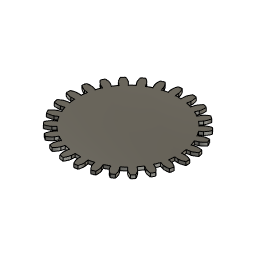
Gear1Finger (Autodesk Fusion 360 design; units mm, degrees)
Autodesk Fusion 360 part; units mm, degrees
sketch "Sketch1" plane through (0, 0, 0) normal (0, 0, 1) x (1, 0, 0)
  spline S0 degree 5 poles (2.4571, -0.2414) (2.4571, -0.2414) (2.4572, -0.2414) (2.4572, -0.2414) (2.4573, -0.2414) (2.4574, -0.2415) (2.4575, -0.2415) (2.4577, -0.2415) (2.4578, -0.2415) (2.458, -0.2415) (2.4582, -0.2415) (2.4584, -0.2415) (2.4586, -0.2415) (2.4589, -0.2416) (2.4591, -0.2416) (2.4594, -0.2416) (2.4597, -0.2416) (2.46, -0.2416) (2.4603, -0.2416) (2.4606, -0.2416) (2.461, -0.2417) (2.4614, -0.2417) (2.4617, -0.2417) (2.4621, -0.2417) (2.4625, -0.2417) (2.463, -0.2417) (2.4634, -0.2417) (2.4639, -0.2417) (2.4643, -0.2418) (2.4648, -0.2418) (2.4653, -0.2418) (2.4658, -0.2418) (2.4664, -0.2418) (2.4669, -0.2418) (2.4675, -0.2418) (2.4681, -0.2418) (2.4686, -0.2418) (2.4692, -0.2418) (2.4699, -0.2418) (2.4705, -0.2418) (2.4712, -0.2418) (2.4718, -0.2418) (2.4725, -0.2418) (2.4732, -0.2418) (2.4739, -0.2418) (2.4746, -0.2417) (2.4754, -0.2417) (2.4761, -0.2417) (2.4769, -0.2417) (2.4777, -0.2417) (2.4785, -0.2416) (2.4793, -0.2416) (2.4801, -0.2416) (2.4809, -0.2415) (2.4818, -0.2415) (2.4826, -0.2415) (2.4835, -0.2414) (2.4844, -0.2414) (2.4853, -0.2413) (2.4862, -0.2413) (2.4872, -0.2412) (2.4881, -0.2412) (2.4891, -0.2411) (2.4901, -0.241) (2.4911, -0.241) (2.4921, -0.2409) (2.4931, -0.2408) (2.4941, -0.2408) (2.4952, -0.2407) (2.4962, -0.2406) (2.4973, -0.2405) (2.4984, -0.2404) (2.4995, -0.2403) (2.5006, -0.2402) (2.5017, -0.2401) (2.5029, -0.24) (2.504, -0.2399) (2.5052, -0.2398) (2.5064, -0.2397) (2.5076, -0.2395) (2.5088, -0.2394) (2.51, -0.2393) (2.5112, -0.2391) (2.5125, -0.239) (2.5137, -0.2388) (2.515, -0.2387) (2.5163, -0.2385) (2.5176, -0.2384) (2.5189, -0.2382) (2.5202, -0.238) (2.5216, -0.2379) (2.5229, -0.2377) (2.5243, -0.2375) (2.5256, -0.2373) (2.527, -0.2371) (2.5284, -0.2369) (2.5298, -0.2367) (2.5313, -0.2365) (2.5327, -0.2363) (2.5341, -0.2361) (2.5356, -0.2358) (2.5371, -0.2356) (2.5386, -0.2354) (2.5401, -0.2351) (2.5416, -0.2349) (2.5431, -0.2346) (2.5446, -0.2344) (2.5462, -0.2341) (2.5477, -0.2338) (2.5493, -0.2336) (2.5509, -0.2333) (2.5525, -0.233) (2.5541, -0.2327) (2.5557, -0.2324) (2.5573, -0.2321) (2.559, -0.2318) (2.5606, -0.2314) (2.5623, -0.2311) (2.564, -0.2308) (2.5657, -0.2304) (2.5674, -0.2301) (2.5691, -0.2297) (2.5708, -0.2294) (2.5725, -0.229) (2.5743, -0.2286) (2.576, -0.2283) (2.5778, -0.2279) (2.5796, -0.2275) (2.5814, -0.2271) (2.5832, -0.2267) (2.585, -0.2263) (2.5868, -0.2258) (2.5886, -0.2254) (2.5905, -0.225) (2.5923, -0.2245) (2.5942, -0.2241) (2.5961, -0.2236) (2.598, -0.2232) (2.5999, -0.2227) (2.6018, -0.2222) (2.6037, -0.2217) (2.6056, -0.2212) (2.6076, -0.2207) (2.6095, -0.2202) (2.6115, -0.2197) (2.6135, -0.2192) (2.6154, -0.2187) (2.6174, -0.2181) (2.6194, -0.2176) (2.6214, -0.217) (2.6235, -0.2165) (2.6255, -0.2159) (2.6275, -0.2153) (2.6296, -0.2147) (2.6317, -0.2141) (2.6337, -0.2135) (2.6358, -0.2129) (2.6379, -0.2123) (2.64, -0.2117) (2.6421, -0.211) (2.6443, -0.2104) (2.6464, -0.2097) (2.6485, -0.2091) (2.6507, -0.2084) (2.6528, -0.2077) (2.655, -0.2071) (2.6572, -0.2064) (2.6594, -0.2057) (2.6616, -0.2049) (2.6638, -0.2042) (2.666, -0.2035) (2.6682, -0.2028) (2.6705, -0.202) (2.6727, -0.2013) (2.675, -0.2005) (2.6772, -0.1997) (2.6795, -0.199) (2.6818, -0.1982) (2.6841, -0.1974) (2.6864, -0.1966) (2.6887, -0.1957) (2.691, -0.1949) (2.6933, -0.1941) (2.6957, -0.1932) (2.698, -0.1924) (2.7004, -0.1915) (2.7027, -0.1907) (2.7051, -0.1898) (2.7075, -0.1889) (2.7099, -0.188) (2.7123, -0.1871) (2.7147, -0.1862) (2.7171, -0.1852) (2.7195, -0.1843) (2.7219, -0.1834) (2.7244, -0.1824) (2.7268, -0.1815) (2.7293, -0.1805) (2.7317, -0.1795) (2.7342, -0.1785) (2.7367, -0.1775) (2.7391, -0.1765) (2.7416, -0.1755) (2.7441, -0.1744) (2.7466, -0.1734) (2.7492, -0.1723) (2.7517, -0.1713) (2.7542, -0.1702) (2.7567, -0.1691) (2.7593, -0.168) (2.7618, -0.1669) (2.7644, -0.1658) (2.767, -0.1647) (2.7695, -0.1636) (2.7721, -0.1624) (2.7747, -0.1613) (2.7773, -0.1601) (2.7799, -0.159) (2.7825, -0.1578) (2.7851, -0.1566) (2.7878, -0.1554) (2.7904, -0.1542) (2.793, -0.153) (2.7957, -0.1517) (2.7983, -0.1505) (2.801, -0.1492) (2.8037, -0.148) (2.8063, -0.1467) (2.809, -0.1454) (2.8117, -0.1441) (2.8144, -0.1428) (2.8171, -0.1415) (2.8198, -0.1402) (2.8225, -0.1388) (2.8252, -0.1375) (2.828, -0.1361) (2.8307, -0.1348) (2.8334, -0.1334) (2.8362, -0.132) (2.8389, -0.1306) (2.8417, -0.1292) (2.8439, -0.128) (2.8455, -0.1272) (2.8466, -0.1266) (2.8472, -0.1263) knots 0 0 0 0 0 0 0.00416667 0.00833333 0.0125 0.01666667 0.02083333 0.025 0.02916667 0.03333333 0.0375 0.04166667 0.04583333 0.05 0.05416667 0.05833333 0.0625 0.06666667 0.07083333 0.075 0.07916667 0.08333333 0.0875 0.09166667 0.09583333 0.1 0.10416667 0.10833333 0.1125 0.11666667 0.12083333 0.125 0.12916667 0.13333333 0.1375 0.14166667 0.14583333 0.15 0.15416667 0.15833333 0.1625 0.16666667 0.17083333 0.175 0.17916667 0.18333333 0.1875 0.19166667 0.19583333 0.2 0.20416667 0.20833333 0.2125 0.21666667 0.22083333 0.225 0.22916667 0.23333333 0.2375 0.24166667 0.24583333 0.25 0.25416667 0.25833333 0.2625 0.26666667 0.27083333 0.275 0.27916667 0.28333333 0.2875 0.29166667 0.29583333 0.3 0.30416667 0.30833333 0.3125 0.31666667 0.32083333 0.325 0.32916667 0.33333333 0.3375 0.34166667 0.34583333 0.35 0.35416667 0.35833333 0.3625 0.36666667 0.37083333 0.375 0.37916667 0.38333333 0.3875 0.39166667 0.39583333 0.4 0.40416667 0.40833333 0.4125 0.41666667 0.42083333 0.425 0.42916667 0.43333333 0.4375 0.44166667 0.44583333 0.45 0.45416667 0.45833333 0.4625 0.46666667 0.47083333 0.475 0.47916667 0.48333333 0.4875 0.49166667 0.49583333 0.5 0.50416667 0.50833333 0.5125 0.51666667 0.52083333 0.525 0.52916667 0.53333333 0.5375 0.54166667 0.54583333 0.55 0.55416667 0.55833333 0.5625 0.56666667 0.57083333 0.575 0.57916667 0.58333333 0.5875 0.59166667 0.59583333 0.6 0.60416667 0.60833333 0.6125 0.61666667 0.62083333 0.625 0.62916667 0.63333333 0.6375 0.64166667 0.64583333 0.65 0.65416667 0.65833333 0.6625 0.66666667 0.67083333 0.675 0.67916667 0.68333333 0.6875 0.69166667 0.69583333 0.7 0.70416667 0.70833333 0.7125 0.71666667 0.72083333 0.725 0.72916667 0.73333333 0.7375 0.74166667 0.74583333 0.75 0.75416667 0.75833333 0.7625 0.76666667 0.77083333 0.775 0.77916667 0.78333333 0.7875 0.79166667 0.79583333 0.8 0.80416667 0.80833333 0.8125 0.81666667 0.82083333 0.825 0.82916667 0.83333333 0.8375 0.84166667 0.84583333 0.85 0.85416667 0.85833333 0.8625 0.86666667 0.87083333 0.875 0.87916667 0.88333333 0.8875 0.89166667 0.89583333 0.9 0.90416667 0.90833333 0.9125 0.91666667 0.92083333 0.925 0.92916667 0.93333333 0.9375 0.94166667 0.94583333 0.95 0.95416667 0.95833333 0.9625 0.96666667 0.97083333 0.975 0.97916667 0.98333333 0.9875 0.99166667 0.99583333 1 1 1 1 1 1
  spline S1 degree 5 poles (2.4571, 0.2414) (2.4571, 0.2414) (2.4572, 0.2414) (2.4572, 0.2414) (2.4573, 0.2414) (2.4574, 0.2415) (2.4575, 0.2415) (2.4577, 0.2415) (2.4578, 0.2415) (2.458, 0.2415) (2.4582, 0.2415) (2.4584, 0.2415) (2.4586, 0.2415) (2.4589, 0.2416) (2.4591, 0.2416) (2.4594, 0.2416) (2.4597, 0.2416) (2.46, 0.2416) (2.4603, 0.2416) (2.4606, 0.2416) (2.461, 0.2417) (2.4614, 0.2417) (2.4617, 0.2417) (2.4621, 0.2417) (2.4625, 0.2417) (2.463, 0.2417) (2.4634, 0.2417) (2.4639, 0.2417) (2.4643, 0.2418) (2.4648, 0.2418) (2.4653, 0.2418) (2.4658, 0.2418) (2.4664, 0.2418) (2.4669, 0.2418) (2.4675, 0.2418) (2.4681, 0.2418) (2.4686, 0.2418) (2.4692, 0.2418) (2.4699, 0.2418) (2.4705, 0.2418) (2.4712, 0.2418) (2.4718, 0.2418) (2.4725, 0.2418) (2.4732, 0.2418) (2.4739, 0.2418) (2.4746, 0.2417) (2.4754, 0.2417) (2.4761, 0.2417) (2.4769, 0.2417) (2.4777, 0.2417) (2.4785, 0.2416) (2.4793, 0.2416) (2.4801, 0.2416) (2.4809, 0.2415) (2.4818, 0.2415) (2.4826, 0.2415) (2.4835, 0.2414) (2.4844, 0.2414) (2.4853, 0.2413) (2.4862, 0.2413) (2.4872, 0.2412) (2.4881, 0.2412) (2.4891, 0.2411) (2.4901, 0.241) (2.4911, 0.241) (2.4921, 0.2409) (2.4931, 0.2408) (2.4941, 0.2408) (2.4952, 0.2407) (2.4962, 0.2406) (2.4973, 0.2405) (2.4984, 0.2404) (2.4995, 0.2403) (2.5006, 0.2402) (2.5017, 0.2401) (2.5029, 0.24) (2.504, 0.2399) (2.5052, 0.2398) (2.5064, 0.2397) (2.5076, 0.2395) (2.5088, 0.2394) (2.51, 0.2393) (2.5112, 0.2391) (2.5125, 0.239) (2.5137, 0.2388) (2.515, 0.2387) (2.5163, 0.2385) (2.5176, 0.2384) (2.5189, 0.2382) (2.5202, 0.238) (2.5216, 0.2379) (2.5229, 0.2377) (2.5243, 0.2375) (2.5256, 0.2373) (2.527, 0.2371) (2.5284, 0.2369) (2.5298, 0.2367) (2.5313, 0.2365) (2.5327, 0.2363) (2.5341, 0.2361) (2.5356, 0.2358) (2.5371, 0.2356) (2.5386, 0.2354) (2.5401, 0.2351) (2.5416, 0.2349) (2.5431, 0.2346) (2.5446, 0.2344) (2.5462, 0.2341) (2.5477, 0.2338) (2.5493, 0.2336) (2.5509, 0.2333) (2.5525, 0.233) (2.5541, 0.2327) (2.5557, 0.2324) (2.5573, 0.2321) (2.559, 0.2318) (2.5606, 0.2314) (2.5623, 0.2311) (2.564, 0.2308) (2.5657, 0.2304) (2.5674, 0.2301) (2.5691, 0.2297) (2.5708, 0.2294) (2.5725, 0.229) (2.5743, 0.2286) (2.576, 0.2283) (2.5778, 0.2279) (2.5796, 0.2275) (2.5814, 0.2271) (2.5832, 0.2267) (2.585, 0.2263) (2.5868, 0.2258) (2.5886, 0.2254) (2.5905, 0.225) (2.5923, 0.2245) (2.5942, 0.2241) (2.5961, 0.2236) (2.598, 0.2232) (2.5999, 0.2227) (2.6018, 0.2222) (2.6037, 0.2217) (2.6056, 0.2212) (2.6076, 0.2207) (2.6095, 0.2202) (2.6115, 0.2197) (2.6135, 0.2192) (2.6154, 0.2187) (2.6174, 0.2181) (2.6194, 0.2176) (2.6214, 0.217) (2.6235, 0.2165) (2.6255, 0.2159) (2.6275, 0.2153) (2.6296, 0.2147) (2.6317, 0.2141) (2.6337, 0.2135) (2.6358, 0.2129) (2.6379, 0.2123) (2.64, 0.2117) (2.6421, 0.211) (2.6443, 0.2104) (2.6464, 0.2097) (2.6485, 0.2091) (2.6507, 0.2084) (2.6528, 0.2077) (2.655, 0.2071) (2.6572, 0.2064) (2.6594, 0.2057) (2.6616, 0.2049) (2.6638, 0.2042) (2.666, 0.2035) (2.6682, 0.2028) (2.6705, 0.202) (2.6727, 0.2013) (2.675, 0.2005) (2.6772, 0.1997) (2.6795, 0.199) (2.6818, 0.1982) (2.6841, 0.1974) (2.6864, 0.1966) (2.6887, 0.1957) (2.691, 0.1949) (2.6933, 0.1941) (2.6957, 0.1932) (2.698, 0.1924) (2.7004, 0.1915) (2.7027, 0.1907) (2.7051, 0.1898) (2.7075, 0.1889) (2.7099, 0.188) (2.7123, 0.1871) (2.7147, 0.1862) (2.7171, 0.1852) (2.7195, 0.1843) (2.7219, 0.1834) (2.7244, 0.1824) (2.7268, 0.1815) (2.7293, 0.1805) (2.7317, 0.1795) (2.7342, 0.1785) (2.7367, 0.1775) (2.7391, 0.1765) (2.7416, 0.1755) (2.7441, 0.1744) (2.7466, 0.1734) (2.7492, 0.1723) (2.7517, 0.1713) (2.7542, 0.1702) (2.7567, 0.1691) (2.7593, 0.168) (2.7618, 0.1669) (2.7644, 0.1658) (2.767, 0.1647) (2.7695, 0.1636) (2.7721, 0.1624) (2.7747, 0.1613) (2.7773, 0.1601) (2.7799, 0.159) (2.7825, 0.1578) (2.7851, 0.1566) (2.7878, 0.1554) (2.7904, 0.1542) (2.793, 0.153) (2.7957, 0.1517) (2.7983, 0.1505) (2.801, 0.1492) (2.8037, 0.148) (2.8063, 0.1467) (2.809, 0.1454) (2.8117, 0.1441) (2.8144, 0.1428) (2.8171, 0.1415) (2.8198, 0.1402) (2.8225, 0.1388) (2.8252, 0.1375) (2.828, 0.1361) (2.8307, 0.1348) (2.8334, 0.1334) (2.8362, 0.132) (2.8389, 0.1306) (2.8417, 0.1292) (2.8439, 0.128) (2.8455, 0.1272) (2.8466, 0.1266) (2.8472, 0.1263) knots 0 0 0 0 0 0 0.00416667 0.00833333 0.0125 0.01666667 0.02083333 0.025 0.02916667 0.03333333 0.0375 0.04166667 0.04583333 0.05 0.05416667 0.05833333 0.0625 0.06666667 0.07083333 0.075 0.07916667 0.08333333 0.0875 0.09166667 0.09583333 0.1 0.10416667 0.10833333 0.1125 0.11666667 0.12083333 0.125 0.12916667 0.13333333 0.1375 0.14166667 0.14583333 0.15 0.15416667 0.15833333 0.1625 0.16666667 0.17083333 0.175 0.17916667 0.18333333 0.1875 0.19166667 0.19583333 0.2 0.20416667 0.20833333 0.2125 0.21666667 0.22083333 0.225 0.22916667 0.23333333 0.2375 0.24166667 0.24583333 0.25 0.25416667 0.25833333 0.2625 0.26666667 0.27083333 0.275 0.27916667 0.28333333 0.2875 0.29166667 0.29583333 0.3 0.30416667 0.30833333 0.3125 0.31666667 0.32083333 0.325 0.32916667 0.33333333 0.3375 0.34166667 0.34583333 0.35 0.35416667 0.35833333 0.3625 0.36666667 0.37083333 0.375 0.37916667 0.38333333 0.3875 0.39166667 0.39583333 0.4 0.40416667 0.40833333 0.4125 0.41666667 0.42083333 0.425 0.42916667 0.43333333 0.4375 0.44166667 0.44583333 0.45 0.45416667 0.45833333 0.4625 0.46666667 0.47083333 0.475 0.47916667 0.48333333 0.4875 0.49166667 0.49583333 0.5 0.50416667 0.50833333 0.5125 0.51666667 0.52083333 0.525 0.52916667 0.53333333 0.5375 0.54166667 0.54583333 0.55 0.55416667 0.55833333 0.5625 0.56666667 0.57083333 0.575 0.57916667 0.58333333 0.5875 0.59166667 0.59583333 0.6 0.60416667 0.60833333 0.6125 0.61666667 0.62083333 0.625 0.62916667 0.63333333 0.6375 0.64166667 0.64583333 0.65 0.65416667 0.65833333 0.6625 0.66666667 0.67083333 0.675 0.67916667 0.68333333 0.6875 0.69166667 0.69583333 0.7 0.70416667 0.70833333 0.7125 0.71666667 0.72083333 0.725 0.72916667 0.73333333 0.7375 0.74166667 0.74583333 0.75 0.75416667 0.75833333 0.7625 0.76666667 0.77083333 0.775 0.77916667 0.78333333 0.7875 0.79166667 0.79583333 0.8 0.80416667 0.80833333 0.8125 0.81666667 0.82083333 0.825 0.82916667 0.83333333 0.8375 0.84166667 0.84583333 0.85 0.85416667 0.85833333 0.8625 0.86666667 0.87083333 0.875 0.87916667 0.88333333 0.8875 0.89166667 0.89583333 0.9 0.90416667 0.90833333 0.9125 0.91666667 0.92083333 0.925 0.92916667 0.93333333 0.9375 0.94166667 0.94583333 0.95 0.95416667 0.95833333 0.9625 0.96666667 0.97083333 0.975 0.97916667 0.98333333 0.9875 0.99166667 0.99583333 1 1 1 1 1 1
  spline S2 degree 5 poles (2.4569, -0.2414) (2.457, -0.2414) (2.457, -0.2414) (2.457, -0.2414) (2.457, -0.2414) (2.457, -0.2414) (2.4571, -0.2414) (2.4571, -0.2414) (2.4571, -0.2414) (2.4571, -0.2414) knots 0 0 0 0 0 0 0.2 0.4 0.6 0.8 1 1 1 1 1 1
  spline S3 degree 5 poles (2.4569, 0.2414) (2.457, 0.2414) (2.457, 0.2414) (2.457, 0.2414) (2.457, 0.2414) (2.457, 0.2414) (2.4571, 0.2414) (2.4571, 0.2414) (2.4571, 0.2414) (2.4571, 0.2414) knots 0 0 0 0 0 0 0.2 0.4 0.6 0.8 1 1 1 1 1 1
  line L0 (0, 0) -> (2.4569, -0.2414)
  line L1 (0, 0) -> (2.4569, 0.2414)
  arc A0 (2.8472, -0.1263) -> (2.8472, 0.1263) centre (0, 0) ccw
  point P0 (2.4576, -0.2415)
  point P1 (2.4585, -0.2415)
  point P2 (2.4597, -0.2416)
  point P3 (2.4612, -0.2417)
  point P4 (2.4631, -0.2417)
  point P5 (2.4653, -0.2418)
  point P6 (2.4679, -0.2418)
  point P7 (2.4708, -0.2418)
  point P8 (2.474, -0.2417)
  point P9 (2.4776, -0.2417)
  point P10 (2.4816, -0.2415)
  point P11 (2.4858, -0.2413)
  point P12 (2.4904, -0.241)
  point P13 (2.4954, -0.2407)
  point P14 (2.5007, -0.2402)
  point P15 (2.5063, -0.2397)
  point P16 (2.5122, -0.239)
  point P17 (2.5185, -0.2383)
  point P18 (2.5251, -0.2374)
  point P19 (2.5321, -0.2364)
  point P20 (2.5393, -0.2352)
  point P21 (2.5469, -0.234)
  point P22 (2.5548, -0.2325)
  point P23 (2.5631, -0.231)
  point P24 (2.5716, -0.2292)
  point P25 (2.5805, -0.2273)
  point P26 (2.5896, -0.2252)
  point P27 (2.5991, -0.2229)
  point P28 (2.6089, -0.2204)
  point P29 (2.619, -0.2177)
  point P30 (2.6294, -0.2148)
  point P31 (2.64, -0.2117)
  point P32 (2.651, -0.2083)
  point P33 (2.6622, -0.2047)
  point P34 (2.6738, -0.2009)
  point P35 (2.6856, -0.1969)
  point P36 (2.6976, -0.1925)
  point P37 (2.71, -0.188)
  point P38 (2.7226, -0.1831)
  point P39 (2.7355, -0.178)
  point P40 (2.7486, -0.1726)
  point P41 (2.762, -0.1669)
  point P42 (2.7756, -0.1609)
  point P43 (2.7895, -0.1546)
  point P44 (2.8036, -0.148)
  point P45 (2.8179, -0.1411)
  point P46 (2.8324, -0.1339)
  point P47 (2.4576, 0.2415)
  point P48 (2.4585, 0.2415)
  point P49 (2.4597, 0.2416)
  point P50 (2.4612, 0.2417)
  point P51 (2.4631, 0.2417)
  point P52 (2.4653, 0.2418)
  point P53 (2.4679, 0.2418)
  point P54 (2.4708, 0.2418)
  point P55 (2.474, 0.2417)
  point P56 (2.4776, 0.2417)
  point P57 (2.4816, 0.2415)
  point P58 (2.4858, 0.2413)
  point P59 (2.4904, 0.241)
  point P60 (2.4954, 0.2407)
  point P61 (2.5007, 0.2402)
  point P62 (2.5063, 0.2397)
  point P63 (2.5122, 0.239)
  point P64 (2.5185, 0.2383)
  point P65 (2.5251, 0.2374)
  point P66 (2.5321, 0.2364)
  point P67 (2.5393, 0.2352)
  point P68 (2.5469, 0.234)
  point P69 (2.5548, 0.2325)
  point P70 (2.5631, 0.231)
  point P71 (2.5716, 0.2292)
  point P72 (2.5805, 0.2273)
  point P73 (2.5896, 0.2252)
  point P74 (2.5991, 0.2229)
  point P75 (2.6089, 0.2204)
  point P76 (2.619, 0.2177)
  point P77 (2.6294, 0.2148)
  point P78 (2.64, 0.2117)
  point P79 (2.651, 0.2083)
  point P80 (2.6622, 0.2047)
  point P81 (2.6738, 0.2009)
  point P82 (2.6856, 0.1969)
  point P83 (2.6976, 0.1925)
  point P84 (2.71, 0.188)
  point P85 (2.7226, 0.1831)
  point P86 (2.7355, 0.178)
  point P87 (2.7486, 0.1726)
  point P88 (2.762, 0.1669)
  point P89 (2.7756, 0.1609)
  point P90 (2.7895, 0.1546)
  point P91 (2.8036, 0.148)
  point P92 (2.8179, 0.1411)
  point P93 (2.8324, 0.1339)
sketch "Sketch2" plane through (0, 0, 0) normal (0, 0, 1) x (1, 0, 0)
  circle A0 centre (0, 0) radius 2.175
combine "Combine1" [no effect]
sketch "Sketch3" plane through (0, 0, 0) normal (0, 0, 1) x (1, 0, 0)
  line L0 (0, 0) -> (48.3149, 0) construction
  line L1 (48.3149, 0) -> (48.3149, 3) construction
  line L2 (48.3149, 3) -> (0, 3) construction
  line L3 (0, 3) -> (0, 0) construction
  constraint perpendicular L0 L1
  constraint parallel L0 L2
  constraint parallel L1 L3
sketch "Sketch4" plane through (0, 0, 0) normal (0, 0, 1) x (1, 0, 0)
  spline S0 degree 5 poles (81.6346, -5.3924) (81.6353, -5.3925) (81.6368, -5.3925) (81.6394, -5.3927) (81.6435, -5.3929) (81.6498, -5.3932) (81.6571, -5.3935) (81.6654, -5.3938) (81.6746, -5.3941) (81.6846, -5.3944) (81.6954, -5.3947) (81.707, -5.395) (81.7193, -5.3953) (81.7323, -5.3955) (81.746, -5.3957) (81.7604, -5.3959) (81.7753, -5.396) (81.7908, -5.3961) (81.807, -5.3961) (81.8236, -5.3961) (81.8408, -5.396) (81.8586, -5.3959) (81.8768, -5.3957) (81.8956, -5.3955) (81.9148, -5.3951) (81.9344, -5.3948) (81.9546, -5.3943) (81.9751, -5.3938) (81.9961, -5.3933) (82.0176, -5.3926) (82.0394, -5.3919) (82.0616, -5.3911) (82.0843, -5.3903) (82.1073, -5.3893) (82.1307, -5.3883) (82.1544, -5.3872) (82.1785, -5.386) (82.203, -5.3848) (82.2278, -5.3835) (82.253, -5.382) (82.2785, -5.3806) (82.3043, -5.379) (82.3305, -5.3773) (82.357, -5.3755) (82.3837, -5.3737) (82.4108, -5.3718) (82.4382, -5.3698) (82.4659, -5.3677) (82.4939, -5.3655) (82.5222, -5.3632) (82.5507, -5.3608) (82.5796, -5.3583) (82.6087, -5.3558) (82.6381, -5.3531) (82.6677, -5.3504) (82.6976, -5.3476) (82.7278, -5.3446) (82.7582, -5.3416) (82.7889, -5.3385) (82.8199, -5.3353) (82.851, -5.332) (82.8825, -5.3285) (82.9141, -5.325) (82.946, -5.3214) (82.9782, -5.3177) (83.0105, -5.3139) (83.0431, -5.31) (83.076, -5.306) (83.109, -5.3019) (83.1423, -5.2977) (83.1757, -5.2935) (83.2094, -5.2891) (83.2434, -5.2846) (83.2775, -5.28) (83.3118, -5.2753) (83.3464, -5.2704) (83.3811, -5.2655) (83.416, -5.2605) (83.4512, -5.2554) (83.4865, -5.2502) (83.5221, -5.2449) (83.5578, -5.2395) (83.5937, -5.234) (83.6298, -5.2283) (83.6661, -5.2226) (83.7026, -5.2168) (83.7393, -5.2108) (83.7761, -5.2048) (83.8131, -5.1986) (83.8503, -5.1924) (83.8877, -5.186) (83.9253, -5.1795) (83.963, -5.1729) (84.0009, -5.1663) (84.0389, -5.1595) (84.0772, -5.1526) (84.1156, -5.1456) (84.1541, -5.1385) (84.1929, -5.1313) (84.2318, -5.1239) (84.2708, -5.1165) (84.31, -5.109) (84.3494, -5.1013) (84.3889, -5.0936) (84.4286, -5.0857) (84.4684, -5.0777) (84.5084, -5.0696) (84.5485, -5.0614) (84.5888, -5.0531) (84.6292, -5.0447) (84.6698, -5.0362) (84.7105, -5.0276) (84.7514, -5.0189) (84.7924, -5.01) (84.8336, -5.0011) (84.8749, -4.992) (84.9163, -4.9828) (84.9579, -4.9735) (84.9996, -4.9641) (85.0414, -4.9546) (85.0834, -4.945) (85.1255, -4.9353) (85.1677, -4.9254) (85.2101, -4.9155) (85.2526, -4.9054) (85.2952, -4.8953) (85.338, -4.885) (85.3809, -4.8746) (85.4239, -4.8641) (85.467, -4.8535) (85.5103, -4.8427) (85.5537, -4.8319) (85.5972, -4.8209) (85.6408, -4.8099) (85.6845, -4.7987) (85.7284, -4.7874) (85.7724, -4.776) (85.8165, -4.7645) (85.8607, -4.7529) (85.905, -4.7411) (85.9495, -4.7293) (85.9941, -4.7173) (86.0387, -4.7053) (86.0835, -4.6931) (86.1284, -4.6808) (86.1734, -4.6684) (86.2185, -4.6558) (86.2638, -4.6432) (86.3091, -4.6305) (86.3545, -4.6176) (86.4001, -4.6046) (86.4457, -4.5915) (86.4915, -4.5783) (86.5374, -4.565) (86.5833, -4.5516) (86.6294, -4.538) (86.6755, -4.5244) (86.7218, -4.5106) (86.7682, -4.4967) (86.8146, -4.4827) (86.8612, -4.4686) (86.9079, -4.4544) (86.9546, -4.4401) (87.0015, -4.4256) (87.0484, -4.4111) (87.0955, -4.3964) (87.1426, -4.3816) (87.1898, -4.3667) (87.2372, -4.3517) (87.2846, -4.3365) (87.3321, -4.3213) (87.3797, -4.3059) (87.4274, -4.2905) (87.4751, -4.2749) (87.523, -4.2592) (87.5709, -4.2433) (87.619, -4.2274) (87.6671, -4.2114) (87.7153, -4.1952) (87.7636, -4.1789) (87.812, -4.1625) (87.8605, -4.146) (87.909, -4.1294) (87.9576, -4.1127) (88.0064, -4.0958) (88.0551, -4.0789) (88.104, -4.0618) (88.153, -4.0446) (88.202, -4.0273) (88.2511, -4.0099) (88.3003, -3.9924) (88.3496, -3.9747) (88.3989, -3.9569) (88.4484, -3.9391) (88.4979, -3.9211) (88.5474, -3.903) (88.5971, -3.8848) (88.6468, -3.8664) (88.6966, -3.848) (88.7465, -3.8294) (88.7964, -3.8107) (88.8464, -3.7919) (88.8965, -3.773) (88.9467, -3.754) (88.9969, -3.7349) (89.0472, -3.7156) (89.0976, -3.6962) (89.148, -3.6768) (89.1985, -3.6572) (89.2491, -3.6374) (89.2998, -3.6176) (89.3505, -3.5977) (89.4012, -3.5776) (89.4521, -3.5575) (89.503, -3.5372) (89.554, -3.5168) (89.605, -3.4963) (89.6561, -3.4756) (89.7073, -3.4549) (89.7585, -3.434) (89.8098, -3.413) (89.8611, -3.392) (89.9126, -3.3708) (89.964, -3.3494) (90.0156, -3.328) (90.0672, -3.3065) (90.1188, -3.2848) (90.1705, -3.263) (90.2223, -3.2411) (90.2741, -3.2191) (90.326, -3.197) (90.378, -3.1748) (90.43, -3.1524) (90.482, -3.1299) (90.5342, -3.1074) (90.5863, -3.0847) (90.6386, -3.0619) (90.6908, -3.0389) (90.7432, -3.0159) (90.7956, -2.9927) (90.848, -2.9695) (90.89, -2.9508) (90.9215, -2.9367) (90.9425, -2.9273) (90.9531, -2.9226) knots 0 0 0 0 0 0 0.00416667 0.00833333 0.0125 0.01666667 0.02083333 0.025 0.02916667 0.03333333 0.0375 0.04166667 0.04583333 0.05 0.05416667 0.05833333 0.0625 0.06666667 0.07083333 0.075 0.07916667 0.08333333 0.0875 0.09166667 0.09583333 0.1 0.10416667 0.10833333 0.1125 0.11666667 0.12083333 0.125 0.12916667 0.13333333 0.1375 0.14166667 0.14583333 0.15 0.15416667 0.15833333 0.1625 0.16666667 0.17083333 0.175 0.17916667 0.18333333 0.1875 0.19166667 0.19583333 0.2 0.20416667 0.20833333 0.2125 0.21666667 0.22083333 0.225 0.22916667 0.23333333 0.2375 0.24166667 0.24583333 0.25 0.25416667 0.25833333 0.2625 0.26666667 0.27083333 0.275 0.27916667 0.28333333 0.2875 0.29166667 0.29583333 0.3 0.30416667 0.30833333 0.3125 0.31666667 0.32083333 0.325 0.32916667 0.33333333 0.3375 0.34166667 0.34583333 0.35 0.35416667 0.35833333 0.3625 0.36666667 0.37083333 0.375 0.37916667 0.38333333 0.3875 0.39166667 0.39583333 0.4 0.40416667 0.40833333 0.4125 0.41666667 0.42083333 0.425 0.42916667 0.43333333 0.4375 0.44166667 0.44583333 0.45 0.45416667 0.45833333 0.4625 0.46666667 0.47083333 0.475 0.47916667 0.48333333 0.4875 0.49166667 0.49583333 0.5 0.50416667 0.50833333 0.5125 0.51666667 0.52083333 0.525 0.52916667 0.53333333 0.5375 0.54166667 0.54583333 0.55 0.55416667 0.55833333 0.5625 0.56666667 0.57083333 0.575 0.57916667 0.58333333 0.5875 0.59166667 0.59583333 0.6 0.60416667 0.60833333 0.6125 0.61666667 0.62083333 0.625 0.62916667 0.63333333 0.6375 0.64166667 0.64583333 0.65 0.65416667 0.65833333 0.6625 0.66666667 0.67083333 0.675 0.67916667 0.68333333 0.6875 0.69166667 0.69583333 0.7 0.70416667 0.70833333 0.7125 0.71666667 0.72083333 0.725 0.72916667 0.73333333 0.7375 0.74166667 0.74583333 0.75 0.75416667 0.75833333 0.7625 0.76666667 0.77083333 0.775 0.77916667 0.78333333 0.7875 0.79166667 0.79583333 0.8 0.80416667 0.80833333 0.8125 0.81666667 0.82083333 0.825 0.82916667 0.83333333 0.8375 0.84166667 0.84583333 0.85 0.85416667 0.85833333 0.8625 0.86666667 0.87083333 0.875 0.87916667 0.88333333 0.8875 0.89166667 0.89583333 0.9 0.90416667 0.90833333 0.9125 0.91666667 0.92083333 0.925 0.92916667 0.93333333 0.9375 0.94166667 0.94583333 0.95 0.95416667 0.95833333 0.9625 0.96666667 0.97083333 0.975 0.97916667 0.98333333 0.9875 0.99166667 0.99583333 1 1 1 1 1 1
  spline S1 degree 5 poles (81.6346, 5.3924) (81.6353, 5.3925) (81.6368, 5.3925) (81.6394, 5.3927) (81.6435, 5.3929) (81.6498, 5.3932) (81.6571, 5.3935) (81.6654, 5.3938) (81.6746, 5.3941) (81.6846, 5.3944) (81.6954, 5.3947) (81.707, 5.395) (81.7193, 5.3953) (81.7323, 5.3955) (81.746, 5.3957) (81.7604, 5.3959) (81.7753, 5.396) (81.7908, 5.3961) (81.807, 5.3961) (81.8236, 5.3961) (81.8408, 5.396) (81.8586, 5.3959) (81.8768, 5.3957) (81.8956, 5.3955) (81.9148, 5.3951) (81.9344, 5.3948) (81.9546, 5.3943) (81.9751, 5.3938) (81.9961, 5.3933) (82.0176, 5.3926) (82.0394, 5.3919) (82.0616, 5.3911) (82.0843, 5.3903) (82.1073, 5.3893) (82.1307, 5.3883) (82.1544, 5.3872) (82.1785, 5.386) (82.203, 5.3848) (82.2278, 5.3835) (82.253, 5.382) (82.2785, 5.3806) (82.3043, 5.379) (82.3305, 5.3773) (82.357, 5.3755) (82.3837, 5.3737) (82.4108, 5.3718) (82.4382, 5.3698) (82.4659, 5.3677) (82.4939, 5.3655) (82.5222, 5.3632) (82.5507, 5.3608) (82.5796, 5.3583) (82.6087, 5.3558) (82.6381, 5.3531) (82.6677, 5.3504) (82.6976, 5.3476) (82.7278, 5.3446) (82.7582, 5.3416) (82.7889, 5.3385) (82.8199, 5.3353) (82.851, 5.332) (82.8825, 5.3285) (82.9141, 5.325) (82.946, 5.3214) (82.9782, 5.3177) (83.0105, 5.3139) (83.0431, 5.31) (83.076, 5.306) (83.109, 5.3019) (83.1423, 5.2977) (83.1757, 5.2935) (83.2094, 5.2891) (83.2434, 5.2846) (83.2775, 5.28) (83.3118, 5.2753) (83.3464, 5.2704) (83.3811, 5.2655) (83.416, 5.2605) (83.4512, 5.2554) (83.4865, 5.2502) (83.5221, 5.2449) (83.5578, 5.2395) (83.5937, 5.234) (83.6298, 5.2283) (83.6661, 5.2226) (83.7026, 5.2168) (83.7393, 5.2108) (83.7761, 5.2048) (83.8131, 5.1986) (83.8503, 5.1924) (83.8877, 5.186) (83.9253, 5.1795) (83.963, 5.1729) (84.0009, 5.1663) (84.0389, 5.1595) (84.0772, 5.1526) (84.1156, 5.1456) (84.1541, 5.1385) (84.1929, 5.1313) (84.2318, 5.1239) (84.2708, 5.1165) (84.31, 5.109) (84.3494, 5.1013) (84.3889, 5.0936) (84.4286, 5.0857) (84.4684, 5.0777) (84.5084, 5.0696) (84.5485, 5.0614) (84.5888, 5.0531) (84.6292, 5.0447) (84.6698, 5.0362) (84.7105, 5.0276) (84.7514, 5.0189) (84.7924, 5.01) (84.8336, 5.0011) (84.8749, 4.992) (84.9163, 4.9828) (84.9579, 4.9735) (84.9996, 4.9641) (85.0414, 4.9546) (85.0834, 4.945) (85.1255, 4.9353) (85.1677, 4.9254) (85.2101, 4.9155) (85.2526, 4.9054) (85.2952, 4.8953) (85.338, 4.885) (85.3809, 4.8746) (85.4239, 4.8641) (85.467, 4.8535) (85.5103, 4.8427) (85.5537, 4.8319) (85.5972, 4.8209) (85.6408, 4.8099) (85.6845, 4.7987) (85.7284, 4.7874) (85.7724, 4.776) (85.8165, 4.7645) (85.8607, 4.7529) (85.905, 4.7411) (85.9495, 4.7293) (85.9941, 4.7173) (86.0387, 4.7053) (86.0835, 4.6931) (86.1284, 4.6808) (86.1734, 4.6684) (86.2185, 4.6558) (86.2638, 4.6432) (86.3091, 4.6305) (86.3545, 4.6176) (86.4001, 4.6046) (86.4457, 4.5915) (86.4915, 4.5783) (86.5374, 4.565) (86.5833, 4.5516) (86.6294, 4.538) (86.6755, 4.5244) (86.7218, 4.5106) (86.7682, 4.4967) (86.8146, 4.4827) (86.8612, 4.4686) (86.9079, 4.4544) (86.9546, 4.4401) (87.0015, 4.4256) (87.0484, 4.4111) (87.0955, 4.3964) (87.1426, 4.3816) (87.1898, 4.3667) (87.2372, 4.3517) (87.2846, 4.3365) (87.3321, 4.3213) (87.3797, 4.3059) (87.4274, 4.2905) (87.4751, 4.2749) (87.523, 4.2592) (87.5709, 4.2433) (87.619, 4.2274) (87.6671, 4.2114) (87.7153, 4.1952) (87.7636, 4.1789) (87.812, 4.1625) (87.8605, 4.146) (87.909, 4.1294) (87.9576, 4.1127) (88.0064, 4.0958) (88.0551, 4.0789) (88.104, 4.0618) (88.153, 4.0446) (88.202, 4.0273) (88.2511, 4.0099) (88.3003, 3.9924) (88.3496, 3.9747) (88.3989, 3.9569) (88.4484, 3.9391) (88.4979, 3.9211) (88.5474, 3.903) (88.5971, 3.8848) (88.6468, 3.8664) (88.6966, 3.848) (88.7465, 3.8294) (88.7964, 3.8107) (88.8464, 3.7919) (88.8965, 3.773) (88.9467, 3.754) (88.9969, 3.7349) (89.0472, 3.7156) (89.0976, 3.6962) (89.148, 3.6768) (89.1985, 3.6572) (89.2491, 3.6374) (89.2998, 3.6176) (89.3505, 3.5977) (89.4012, 3.5776) (89.4521, 3.5575) (89.503, 3.5372) (89.554, 3.5168) (89.605, 3.4963) (89.6561, 3.4756) (89.7073, 3.4549) (89.7585, 3.434) (89.8098, 3.413) (89.8611, 3.392) (89.9126, 3.3708) (89.964, 3.3494) (90.0156, 3.328) (90.0672, 3.3065) (90.1188, 3.2848) (90.1705, 3.263) (90.2223, 3.2411) (90.2741, 3.2191) (90.326, 3.197) (90.378, 3.1748) (90.43, 3.1524) (90.482, 3.1299) (90.5342, 3.1074) (90.5863, 3.0847) (90.6386, 3.0619) (90.6908, 3.0389) (90.7432, 3.0159) (90.7956, 2.9927) (90.848, 2.9695) (90.89, 2.9508) (90.9215, 2.9367) (90.9425, 2.9273) (90.9531, 2.9226) knots 0 0 0 0 0 0 0.00416667 0.00833333 0.0125 0.01666667 0.02083333 0.025 0.02916667 0.03333333 0.0375 0.04166667 0.04583333 0.05 0.05416667 0.05833333 0.0625 0.06666667 0.07083333 0.075 0.07916667 0.08333333 0.0875 0.09166667 0.09583333 0.1 0.10416667 0.10833333 0.1125 0.11666667 0.12083333 0.125 0.12916667 0.13333333 0.1375 0.14166667 0.14583333 0.15 0.15416667 0.15833333 0.1625 0.16666667 0.17083333 0.175 0.17916667 0.18333333 0.1875 0.19166667 0.19583333 0.2 0.20416667 0.20833333 0.2125 0.21666667 0.22083333 0.225 0.22916667 0.23333333 0.2375 0.24166667 0.24583333 0.25 0.25416667 0.25833333 0.2625 0.26666667 0.27083333 0.275 0.27916667 0.28333333 0.2875 0.29166667 0.29583333 0.3 0.30416667 0.30833333 0.3125 0.31666667 0.32083333 0.325 0.32916667 0.33333333 0.3375 0.34166667 0.34583333 0.35 0.35416667 0.35833333 0.3625 0.36666667 0.37083333 0.375 0.37916667 0.38333333 0.3875 0.39166667 0.39583333 0.4 0.40416667 0.40833333 0.4125 0.41666667 0.42083333 0.425 0.42916667 0.43333333 0.4375 0.44166667 0.44583333 0.45 0.45416667 0.45833333 0.4625 0.46666667 0.47083333 0.475 0.47916667 0.48333333 0.4875 0.49166667 0.49583333 0.5 0.50416667 0.50833333 0.5125 0.51666667 0.52083333 0.525 0.52916667 0.53333333 0.5375 0.54166667 0.54583333 0.55 0.55416667 0.55833333 0.5625 0.56666667 0.57083333 0.575 0.57916667 0.58333333 0.5875 0.59166667 0.59583333 0.6 0.60416667 0.60833333 0.6125 0.61666667 0.62083333 0.625 0.62916667 0.63333333 0.6375 0.64166667 0.64583333 0.65 0.65416667 0.65833333 0.6625 0.66666667 0.67083333 0.675 0.67916667 0.68333333 0.6875 0.69166667 0.69583333 0.7 0.70416667 0.70833333 0.7125 0.71666667 0.72083333 0.725 0.72916667 0.73333333 0.7375 0.74166667 0.74583333 0.75 0.75416667 0.75833333 0.7625 0.76666667 0.77083333 0.775 0.77916667 0.78333333 0.7875 0.79166667 0.79583333 0.8 0.80416667 0.80833333 0.8125 0.81666667 0.82083333 0.825 0.82916667 0.83333333 0.8375 0.84166667 0.84583333 0.85 0.85416667 0.85833333 0.8625 0.86666667 0.87083333 0.875 0.87916667 0.88333333 0.8875 0.89166667 0.89583333 0.9 0.90416667 0.90833333 0.9125 0.91666667 0.92083333 0.925 0.92916667 0.93333333 0.9375 0.94166667 0.94583333 0.95 0.95416667 0.95833333 0.9625 0.96666667 0.97083333 0.975 0.97916667 0.98333333 0.9875 0.99166667 0.99583333 1 1 1 1 1 1
  spline S2 degree 5 poles (81.6306, -5.3922) (81.6307, -5.3922) (81.6311, -5.3922) (81.6315, -5.3922) (81.6322, -5.3923) (81.633, -5.3923) (81.6336, -5.3924) (81.6341, -5.3924) (81.6345, -5.3924) (81.6346, -5.3924) knots 0 0 0 0 0 0 0.2 0.4 0.6 0.8 1 1 1 1 1 1
  spline S3 degree 5 poles (81.6306, 5.3922) (81.6307, 5.3922) (81.6311, 5.3922) (81.6315, 5.3922) (81.6322, 5.3923) (81.633, 5.3923) (81.6336, 5.3924) (81.6341, 5.3924) (81.6345, 5.3924) (81.6346, 5.3924) knots 0 0 0 0 0 0 0.2 0.4 0.6 0.8 1 1 1 1 1 1
  line L0 (0, 0) -> (81.6306, -5.3922)
  line L1 (0, 0) -> (81.6306, 5.3922)
  arc A0 (90.9531, -2.9226) -> (90.9531, 2.9226) centre (0, 0) ccw
  point P0 (81.6467, -5.393)
  point P1 (81.6669, -5.3939)
  point P2 (81.6952, -5.3947)
  point P3 (81.7316, -5.3955)
  point P4 (81.7761, -5.396)
  point P5 (81.8286, -5.3961)
  point P6 (81.8893, -5.3955)
  point P7 (81.958, -5.3942)
  point P8 (82.0348, -5.3921)
  point P9 (82.1196, -5.3888)
  point P10 (82.2125, -5.3843)
  point P11 (82.3134, -5.3784)
  point P12 (82.4223, -5.3709)
  point P13 (82.5392, -5.3618)
  point P14 (82.6641, -5.3507)
  point P15 (82.7969, -5.3376)
  point P16 (82.9376, -5.3224)
  point P17 (83.0861, -5.3048)
  point P18 (83.2425, -5.2846)
  point P19 (83.4067, -5.2619)
  point P20 (83.5787, -5.2363)
  point P21 (83.7584, -5.2077)
  point P22 (83.9457, -5.1759)
  point P23 (84.1407, -5.1409)
  point P24 (84.3433, -5.1025)
  point P25 (84.5535, -5.0604)
  point P26 (84.7711, -5.0146)
  point P27 (84.9961, -4.9649)
  point P28 (85.2285, -4.9111)
  point P29 (85.4682, -4.8531)
  point P30 (85.7152, -4.7908)
  point P31 (85.9694, -4.724)
  point P32 (86.2307, -4.6524)
  point P33 (86.499, -4.5761)
  point P34 (86.7743, -4.4949)
  point P35 (87.0566, -4.4085)
  point P36 (87.3457, -4.3169)
  point P37 (87.6415, -4.2199)
  point P38 (87.944, -4.1174)
  point P39 (88.2531, -4.0092)
  point P40 (88.5687, -3.8951)
  point P41 (88.8908, -3.7752)
  point P42 (89.2192, -3.6491)
  point P43 (89.5538, -3.5168)
  point P44 (89.8946, -3.3781)
  point P45 (90.2415, -3.233)
  point P46 (90.5944, -3.0811)
  point P47 (81.6467, 5.393)
  point P48 (81.6669, 5.3939)
  point P49 (81.6952, 5.3947)
  point P50 (81.7316, 5.3955)
  point P51 (81.7761, 5.396)
  point P52 (81.8286, 5.3961)
  point P53 (81.8893, 5.3955)
  point P54 (81.958, 5.3942)
  point P55 (82.0348, 5.3921)
  point P56 (82.1196, 5.3888)
  point P57 (82.2125, 5.3843)
  point P58 (82.3134, 5.3784)
  point P59 (82.4223, 5.3709)
  point P60 (82.5392, 5.3618)
  point P61 (82.6641, 5.3507)
  point P62 (82.7969, 5.3376)
  point P63 (82.9376, 5.3224)
  point P64 (83.0861, 5.3048)
  point P65 (83.2425, 5.2846)
  point P66 (83.4067, 5.2619)
  point P67 (83.5787, 5.2363)
  point P68 (83.7584, 5.2077)
  point P69 (83.9457, 5.1759)
  point P70 (84.1407, 5.1409)
  point P71 (84.3433, 5.1025)
  point P72 (84.5535, 5.0604)
  point P73 (84.7711, 5.0146)
  point P74 (84.9961, 4.9649)
  point P75 (85.2285, 4.9111)
  point P76 (85.4682, 4.8531)
  point P77 (85.7152, 4.7908)
  point P78 (85.9694, 4.724)
  point P79 (86.2307, 4.6524)
  point P80 (86.499, 4.5761)
  point P81 (86.7743, 4.4949)
  point P82 (87.0566, 4.4085)
  point P83 (87.3457, 4.3169)
  point P84 (87.6415, 4.2199)
  point P85 (87.944, 4.1174)
  point P86 (88.2531, 4.0092)
  point P87 (88.5687, 3.8951)
  point P88 (88.8908, 3.7752)
  point P89 (89.2192, 3.6491)
  point P90 (89.5538, 3.5168)
  point P91 (89.8946, 3.3781)
  point P92 (90.2415, 3.233)
  point P93 (90.5944, 3.0811)
sketch "Sketch5" plane through (0, 0, 0) normal (0, 0, 1) x (1, 0, 0)
  circle A0 centre (0, 0) radius 76.375
extrude "Extrude3" add sketch "Sketch5" along normal blind 5 makes body 1
extrude "Extrude4" add sketch "Sketch4" along normal blind 5 separate body makes body 2
pattern_circular "C-Pattern2" count 26 over 360 about axis through (0, 0, 1.75) along (0, 0, 1) of "Extrude4" makes body 3 makes body 4 makes body 5 makes body 6 makes body 7 makes body 8 makes body 9 makes body 10 makes body 11 makes body 12 makes body 13 makes body 14 makes body 15 makes body 16 makes body 17 makes body 18 makes body 19 makes body 20 makes body 21 makes body 22 makes body 23 makes body 24 makes body 25 makes body 26 makes body 27
combine "Combine2" operation add target body 1 tool bodies 2 3 4 5 6 7 8 9 10 11 12 13 14 15 16 17 18 19 20 21 22 23 24 25 26 27
sketch "Sketch6" plane through (0, 0, 0) normal (0, 0, 1) x (1, 0, 0)
  line L0 (0, 0) -> (48.3413, 0) construction
  line L1 (48.3413, 0) -> (48.3413, 3) construction
  line L2 (48.3413, 3) -> (0, 3) construction
  line L3 (0, 3) -> (0, 0) construction
  constraint perpendicular L0 L1
  constraint parallel L0 L2
  constraint parallel L1 L3
scale "Scale1" factor 1.24911 about (60.3814, -46.7678, 5) bodies 1
scale "Scale2" factor 0.114426 about (48.4246, -68.4395, 5) bodies 1
